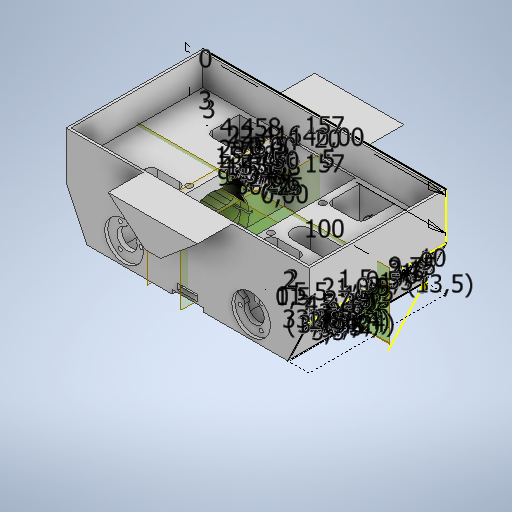
# Autodesk Inventor part: low_part
Saved by Autodesk Inventor 2025 (Build 290162000, 162)
## iProperties
Created: 2026-06-26
Part Number: low_part
Material: Типовые
Document SubType Name: Sheet Metal
Designer: garin
Density: 1 g/cm^3
Appearance: По умолчанию
Sheet Metal Rule: По умолчанию
Mass: 239.505 g
Surface Area: 434.405 cm^2
Volume: 239.505 cm^3
Author: garin
Autodesk Inventor part; units mm, degrees
(part 1 of 2)
ref_plane "YZ Plane" through (0, 0, 0) normal (1, 0, 0) x (0, 1, 0)
ref_plane "XZ Plane" through (0, 0, 0) normal (0, 1, 0) x (-1, 0, 0)
ref_plane "XY Plane" through (0, 0, 0) normal (0, 0, 1) x (1, 0, 0)
sketch "Эскиз2" plane through (0, 0, 0) normal (0, 0, 1) x (1, 0, 0)
  line L0 (0, 0) -> (-78.5, 0) construction
  line L1 (-78.5, 0) -> (78.5, 0)
  line L2 (0, 0) -> (-50, 0) construction
  line L3 (-50, 0) -> (-50, -28.5) construction
  line L4 (-50, -28.5) -> (-78.5, 0)
  line L5 (-50, -28.5) -> (50, -28.5)
  line L6 (50, -28.5) -> (78.5, 0)
  line L7 (-50, -28.5) -> (-45.542, -28.5) construction
  line L8 (-45.542, -28.5) -> (-45.542, -22.152) construction
  line L9 (-45.542, -22.152) -> (-50, -22.152) construction
  line L10 (-50, -22.152) -> (-50, -28.5) construction
  line L11 (-45.542, -22.152) -> (-45.542, -6.564) construction
  arc A0 (-45.542, -22.152) -> (-45.542, -6.564) centre (-50.0424, -14.358) ccw construction
  circle A1 centre (-45.542, -22.152) radius 1.3
  line L12 (-45.542, -22.152) -> (-32.0424, -14.358) construction
  line L13 (-45.542, -22.152) -> (-29.954, -22.152) construction
  circle A2 centre (-32.0424, -14.358) radius 1.3
  circle A3 centre (-45.542, -6.564) radius 1.3
  line L14 (-45.542, -6.564) -> (-32.0424, -14.358) construction
  circle A4 centre (-41.0424, -14.358) radius 12.5
  circle A5 centre (-41.0424, -14.358) radius 6.5
  line L15 (-41.0424, -14.358) -> (-41.0424, -26.858) construction
  line L16 (-41.0424, -14.358) -> (-34.7924, -25.1833) construction
  line L17 (-41.0424, -14.358) -> (-30.2171, -20.608) construction
  line L18 (-78.5, 0) -> (-75.5, 0) construction
  line L19 (-50, -28.5) -> (-47, -28.5) construction
  line L20 (-75.5, 0) -> (-47, -28.5)
  line L21 (-78.5, 0) -> (-75.5, 0) construction
  line L22 (-75.5, 0) -> (-75.5, -3) construction
  line L23 (-75.5, -3) -> (-78.5, -3) construction
  line L24 (-78.5, -3) -> (-78.5, 0) construction
  line L25 (-50, -28.5) -> (-50, -25.5) construction
  line L26 (-50, -28.5) -> (-47, -28.5) construction
  line L27 (-75.5, -3) -> (75.5, -3)
  line L28 (-75.5, -3) -> (75.5, -3) construction
  line L29 (0, 0) -> (0, -28.5) construction
  line L30 (75.5, 0) -> (47, -28.5)
  line L31 (-50, -25.5) -> (50, -25.5)
  line L32 (-50, -25.5) -> (50, -25.5) construction
  circle A6 centre (45.542, -22.152) radius 1.3
  circle A7 centre (32.0424, -14.358) radius 1.3
  circle A8 centre (45.542, -6.564) radius 1.3
  circle A9 centre (41.0424, -14.358) radius 12.5
  circle A10 centre (41.0424, -14.358) radius 6.5
  line L33 (41.0424, -14.358) -> (41.0424, -26.858) construction
  line L34 (41.0424, -14.358) -> (30.2171, -20.608) construction
  line L35 (-41.0424, -14.358) -> (-22.0786, -14.358) construction
  line L36 (-41.0424, -14.358) -> (-41.0424, -1.858)
  line L37 (-41.0424, -14.358) -> (-30.2171, -8.108)
  line L38 (41.0424, -14.358) -> (30.2171, -8.108)
  line L39 (41.0424, -14.358) -> (41.0424, -1.858)
  line L40 (-45.542, -6.564) -> (-50, -6.564) construction
  line L41 (-50, -6.564) -> (-50, 0) construction
  line L42 (-50, 0) -> (-45.542, 0) construction
  line L43 (-45.542, 0) -> (-45.542, -6.564) construction
  line L44 (-50, -25.5) -> (-27.584, -25.5)
  line L45 (-27.584, -25.5) -> (-27.584, 0)
  line L46 (-27.584, 0) -> (-50, 0)
  line L47 (-50, 0) -> (-50, -25.5)
  line L48 (27.584, -25.5) -> (27.584, 0)
  line L49 (50, 0) -> (50, -25.5)
  line L50 (-50, -28.5) -> (-65, -28.5)
  line L51 (-65, -28.5) -> (-78.5, 0)
  line L52 (-65, -28.5) -> (-62, -28.5)
  line L53 (-62, -28.5) -> (-75.5, 0)
  line L54 (-50, -25.5) -> (-63.4211, -25.5)
  line L55 (50, -28.5) -> (65, -28.5)
  line L56 (65, -28.5) -> (78.5, 0)
  line L57 (65, -28.5) -> (62, -28.5)
  line L58 (62, -28.5) -> (75.5, 0)
  point P0 (-72.5, -3)
  point P1 (72.5, -3)
  point P2 (-41.0424, -25.5)
  point P3 (-41.0424, -20.858)
  point P4 (-35.4132, -17.608)
  point P5 (-30.2171, -20.608)
  point P6 (-35.3762, -25.5)
  point P7 (35.3762, -25.5)
  point P8 (30.2171, -20.608)
  point P9 (35.4132, -17.608)
  point P10 (41.0424, -20.858)
  point P11 (41.0424, -25.5)
  point P12 (47, -28.5)
  point P13 (46.7086, -25.5)
  point P14 (41.0424, -26.858)
  point P15 (-46.7086, -25.5)
  point P16 (35.8226, -3)
  point P17 (41.0424, -3)
  point P18 (41.0424, -7.858)
  point P19 (35.4132, -11.108)
  point P20 (30.2171, -8.108)
  point P21 (-35.8226, -3)
  point P22 (-30.2171, -8.108)
  point P23 (-35.4132, -11.108)
  point P24 (-41.0424, -7.858)
  point P25 (-41.0424, -3)
  dimension "d0" = 78.5
  dimension "d1" = 157
  dimension "d2" = 50
  dimension "d3" = 28.5
  dimension "d4" = 100
  dimension "d15" = 4.458
  dimension "d16" = 6.348
  dimension "d17" = 15.588
  dimension "d18" = 9
  dimension "d19" = 2.6
  dimension "d20" = 15.588
  dimension "d21" = 30
  dimension "d22" = 2.6
  dimension "d23" = 2.6
  dimension "d24" = 25
  dimension "d25" = 13
  dimension "d26" = 12.5
  dimension "d29" = 30
  dimension "d31" = 3
  dimension "d32" = 3
  dimension "d33" = 3
  dimension "d34" = 90
  dimension "d35" = 0
  dimension "d36" = 0
  dimension "d48" = 4.458
  dimension "d49" = 22.416
  dimension "d151" = 15
  dimension "d152" = 3
  dimension "d153" = 15
  dimension "d154" = 3
  constraints: 118 end point, 17 symmetric about line, 13 point on line, 12 horizontal, 11 centre point, 9 parallel, 6 coincident, 5 perpendicular, 4 equal length, 3 point on circle, 3 vertical, 1 midpoint, 9 other
  measures "d0" distance of L0.start L0.end
  measures "d1" distance of L0.end L1.end
  measures "d2" distance of L0.start L2.end
  measures "d3" distance of L2.end L3.end
  measures "d4" distance of L3.end L5.end
  measures "d15" distance of L9.end L8.end
  measures "d16" distance of L8.end L7.end
  measures "d17" distance of L8.end L11.end
  measures "d18" radius of A0
  measures "d19" diameter of A1
  measures "d20" distance of L12.start L12.end
  measures "d21" angle of L13 L12
  measures "d22" diameter of A2
  measures "d23" diameter of A3
  measures "d24" diameter of A4
  measures "d25" diameter of A5
  measures "d26" distance of L15.start L15.end
  measures "d31" distance of L0.end L18.end
  measures "d32" distance of L3.end L19.end
  measures "d33" distance of L21.end L22.end
  measures "d34" angle of L26 L25
  measures "d35" distance between parallel lines of L27 L28
  measures "d36" distance between parallel lines of L31 L32
  measures "d48" distance of L41.end L42.end
  measures "d49" distance of L46.end L45.end
  measures "d151" distance of L3.end L50.end
  measures "d152" distance of L50.end L52.end
  measures "d153" distance of L5.end L55.end
  measures "d154" distance of L55.end L57.end
extrude "Выдавливание1" add sketch "Эскиз2" along normal blind 88.4 contours L1 L53 L27 L4 | L4 L53 L50 L51 | L1 L47 L27 L20 | L20 L27 L53 | L27 L53 L4 | L1 L45 L27 A4 L47 | L27 L47 A4 L20 | L20 L54 L4 L53 L27 | L4 L54 L53 | L53 L54 L4 L50 | L1 L48 L27 L45 | L27 A4 L47 | L31 A4 A9 L30 L5 L20 | L47 A4 L31 | L20 L5 L4 L54 | L1 L49 L27 A9 L48 | L45 L31 A4 L27 | L27 L48 L31 L45 | L27 L36 A5 L37 A4 L31 L47 | A4 L36 L27 | L47 A4 | L31 A4 | L1 L30 L27 L49 | L27 A9 L31 L48 | L27 L36 A4 | A4 L37 A5 L36 L27 | L30 L27 L58 L6 L5 | L58 L27 L30 | L1 L6 L27 L58 | L49 A9 L27 | L27 L30 L49 A9 | A9 L39 L27 | L27 L39 A10 L38 A9 | L36 L37 A5 | A5 L37 L36 | L6 L58 L55 | L31 A9 L49 | L56 L55 L58 L6 | L27 L6 L58 | A9 L49 L31 L38 A10 L39 L27 | L27 L39 A9 | A9 L49 | L31 A9 | L39 L38 A10 | A10 L38 L39 | A1 | A2 | A3 | A6 | A7 | A8
extrude "Выдавливание2" cut sketch "Эскиз2" along normal blind 5 contours A4 L37 A5 L36 L27 | L27 L39 A10 L38 A9 | L36 L37 A5 | A5 L37 L36 | L39 L38 A10 | A10 L38 L39 | A1 | A2 | A3 | A6 | A7 | A8
extrude "Выдавливание4" cut sketch "Эскиз2" along normal blind 2 contours L27 L36 A5 L37 A4 L31 L47 | A4 L36 L27 | L47 A4 | L31 A4 | L27 L36 A4 | A4 L37 A5 L36 L27 | A9 L39 L27 | L27 L39 A10 L38 A9 | L36 L37 A5 | A5 L37 L36 | A9 L49 L31 L38 A10 L39 L27 | L27 L39 A9 | A9 L49 | L31 A9 | L39 L38 A10 | A10 L38 L39 | A1 | A2 | A3 | A6 | A7 | A8
fillet "Сопряжение1" radius 2 4 edges at (35.4132, -11.108, 3.5) (41.0424, -7.858, 3.5) (-35.4132, -11.108, 3.5) (-41.0424, -7.858, 3.5)
extrude "Выдавливание6" cut sketch "Эскиз2" along normal blind 21.5 from surface at 5 contours L1 L45 L27 A4 L47 | L27 A4 L47 | L47 A4 L31 | L1 L49 L27 A9 L48 | L45 L31 A4 L27 | L27 L36 A5 L37 A4 L31 L47 | A4 L36 L27 | L27 A9 L31 L48 | L27 L36 A4 | A4 L37 A5 L36 L27 | L49 A9 L27 | A9 L39 L27 | L27 L39 A10 L38 A9 | L36 L37 A5 | A5 L37 L36 | L31 A9 L49 | A9 L49 L31 L38 A10 L39 L27 | L27 L39 A9 | L39 L38 A10 | A10 L38 L39 | A1 | A2 | A3 | A6 | A7 | A8
fillet "Сопряжение2" radius 4 4 edges at (50, -12.75, 26.5) (27.584, -12.75, 26.5) (-27.584, -12.75, 26.5) (-50, -12.75, 26.5)
ref_plane "РабПлоскость1" through (0, 0, 44.2) normal (0, 0, -1) x (-1, 0, 0)
mirror "Зеркальное отражение2" about plane through (0, 0, 44.2) normal (0, 0, -1) of "Выдавливание2", "Выдавливание6", "Сопряжение2", "Выдавливание4", "Сопряжение1"
sketch "Эскиз4" plane through (-78.5, 0, 0) normal (0, 1, 0) x (1, 0, 0)
  line L0 (78.5, 0) -> (78.5, -86) construction
  line L1 (28.5, -86) -> (128.5, -86) projected
  line L2 (0, 0) -> (0, -88.4) projected
  line L3 (0, -44.2) -> (157, -44.2) construction
  line L4 (157, 0) -> (157, -88.4) projected
  line L5 (78.5, -44.2) -> (101.4, -44.2) construction
  line L6 (101.4, -44.2) -> (101.4, -3) construction
  line L7 (101.4, -3) -> (78.5, -3) construction
  line L8 (78.5, -3) -> (78.5, -44.2) construction
  line L9 (101.4, -3) -> (55.6, -3)
  line L10 (55.6, -3) -> (55.6, -85.4)
  line L11 (55.6, -85.4) -> (101.4, -85.4)
  line L12 (101.4, -85.4) -> (101.4, -3)
  dimension "d53" = 22.9
  dimension "d54" = 41.2
  dimension "d55" = 45.8
  dimension "d56" = 82.4
  constraints: 20 end point, 4 midpoint, 4 parallel, 2 horizontal, 2 perpendicular
  measures "d53" distance of L7.end L6.end
  measures "d54" distance of L6.end L5.end
  measures "d55" distance of L11.end L10.end
  measures "d56" distance of L10.end L9.end
extrude "Выдавливание7" cut sketch "Эскиз4" against normal blind 28.5
sketch "Эскиз5" plane through (-78.5, 0, 0) normal (0, 1, 0) x (1, 0, 0)
  line L0 (0, 0) -> (157, 0)
  line L1 (157, 0) -> (157, -88.4)
  line L2 (157, -88.4) -> (0, -88.4)
  line L3 (0, -88.4) -> (0, 0)
  line L4 (55.6, -3) -> (101.4, -3) projected
  line L5 (55.6, -3) -> (55.6, -83) projected
  line L6 (101.4, -3) -> (55.6, -3)
  line L7 (55.6, -3) -> (55.6, -83)
  line L8 (55.6, -83) -> (101.4, -83)
  line L9 (101.4, -83) -> (101.4, -3)
  line L10 (104.4, 0) -> (52.6, 0)
  line L11 (52.6, 0) -> (52.6, -86)
  line L12 (52.6, -86) -> (104.4, -86)
  line L13 (104.4, -86) -> (104.4, 0)
  line L14 (3, -85.4) -> (154, -85.4)
  line L15 (154, -85.4) -> (154, -3)
  line L16 (154, -3) -> (3, -3)
  line L17 (3, -3) -> (3, -85.4)
  line L18 (104.4, 0) -> (106.084, 0)
  line L19 (106.084, 0) -> (106.084, -88.4)
  line L20 (106.084, -88.4) -> (104.4, -88.4)
  line L21 (104.4, -88.4) -> (104.4, 0)
  line L22 (52.6, 0) -> (50.916, 0)
  line L23 (50.916, 0) -> (50.916, -88.4)
  line L24 (50.916, -88.4) -> (52.6, -88.4)
  line L25 (52.6, -88.4) -> (52.6, 0)
  line L26 (50.916, 0) -> (52.916, 0) construction
  line L27 (0, -44.2) -> (157, -44.2) construction
  line L28 (78.5, -86) -> (78.5, 0) construction
  arc A0 (28.5, -22.5) -> (32.5, -26.5) centre (32.5, -22.5) ccw projected
  line L29 (46.916, -26.5) -> (32.5, -26.5) projected
  arc A1 (46.916, -26.5) -> (50.916, -22.5) centre (46.916, -22.5) ccw projected
  line L30 (50.916, -5) -> (50.916, -22.5) projected
  line L31 (50.916, -5) -> (28.5, -5) projected
  line L32 (28.5, -5) -> (28.5, -22.5) projected
  arc A2 (32.5, -61.9) -> (28.5, -65.9) centre (32.5, -65.9) ccw projected
  line L33 (28.5, -83.4) -> (28.5, -65.9) projected
  line L34 (50.916, -83.4) -> (28.5, -83.4) projected
  line L35 (50.916, -83.4) -> (50.916, -65.9) projected
  arc A3 (50.916, -65.9) -> (46.916, -61.9) centre (46.916, -65.9) ccw projected
  line L36 (46.916, -61.9) -> (32.5, -61.9) projected
  arc A4 (110.084, -61.9) -> (106.084, -65.9) centre (110.084, -65.9) ccw projected
  line L37 (106.084, -83.4) -> (106.084, -65.9) projected
  line L38 (128.5, -83.4) -> (106.084, -83.4) projected
  line L39 (128.5, -83.4) -> (128.5, -65.9) projected
  arc A5 (128.5, -65.9) -> (124.5, -61.9) centre (124.5, -65.9) ccw projected
  line L40 (124.5, -61.9) -> (110.084, -61.9) projected
  arc A6 (106.084, -22.5) -> (110.084, -26.5) centre (110.084, -22.5) ccw projected
  line L41 (124.5, -26.5) -> (110.084, -26.5) projected
  arc A7 (124.5, -26.5) -> (128.5, -22.5) centre (124.5, -22.5) ccw projected
  line L42 (128.5, -5) -> (128.5, -22.5) projected
  line L43 (128.5, -5) -> (106.084, -5) projected
  line L44 (106.084, -5) -> (106.084, -22.5) projected
  line L45 (46.916, -61.9) -> (55.6, -61.9) construction
  arc A8 (50.916, -65.9) -> (46.916, -61.9) centre (46.916, -65.9) ccw construction
  line L46 (46.916, -26.5) -> (55.6, -26.5) construction
  line L47 (55.6, -61.9) -> (52.1, -61.9) construction
  line L48 (52.1, -61.9) -> (52.1, -60.9) construction
  line L49 (52.1, -60.9) -> (55.6, -60.9) construction
  line L50 (55.6, -60.9) -> (55.6, -61.9) construction
  circle A9 centre (52.1, -60.9) radius 2.1
  circle A10 centre (52.1, -27.5) radius 2.1
  circle A11 centre (104.9, -60.9) radius 2.1
  circle A12 centre (104.9, -27.5) radius 2.1
  line L51 (101.4, -83) -> (55.6, -83)
  line L52 (55.6, -83) -> (55.6, -85.4)
  line L53 (55.6, -85.4) -> (101.4, -85.4)
  line L54 (101.4, -85.4) -> (101.4, -83)
  point P0 (50.916, -65.9)
  point P1 (50.916, -22.5)
  point P2 (50.916, -83.4)
  point P3 (106.084, -83.4)
  dimension "d59" = 157
  dimension "d60" = 88.4
  dimension "d61" = 3
  dimension "d62" = 3
  dimension "d63" = 1.684
  dimension "d64" = 1.684
  dimension "d72" = 3.5
  dimension "d73" = 1
  dimension "d74" = 4.2
  constraints: 74 end point, 16 parallel, 10 perpendicular, 7 horizontal, 5 point on line, 4 centre point, 3 midpoint, 3 symmetric about line, 3 tangent, 1 coincident, 1 vertical, 9 other
  measures "d59" distance of L1.end L2.end
  measures "d60" distance of L0.end L1.end
  measures "d61" distance between parallel lines of L9 L13
  measures "d62" distance between parallel lines of L2 L14
  measures "d63" distance of L19.end L20.end
  measures "d64" distance of L24.end L23.end
  measures "d72" distance of L48.end L49.end
  measures "d73" distance of L47.end L48.end
  measures "d74" diameter of A9
extrude "Выдавливание8" add sketch "Эскиз5" along normal blind 10.2 contours L0 L23 L16 L17 L14 L2 L3 | L0 L11 L16 L23 | L0 L13 L16 L4 L11 | L23 L31 L32 A0 L29 A1 A10 A9 A3 L36 A2 L33 L34 L14 L17 L16 | L16 L11 A10 L23 | L23 L14 L11 L25 L2 | L0 L19 L16 L13 | L16 L5 L52 L14 L11 A9 A10 | L25 L12 L21 L2 | L23 A9 L11 L14 | L0 L1 L2 L19 L14 L15 L16 | L16 L19 A12 L13 | L13 A12 A11 L14 L54 L9 L16 | L21 L13 L14 L19 L2 | L11 L14 L13 L12 | L16 L15 L14 L19 L38 L39 A5 L40 A4 A11 A12 A6 L41 A7 L42 L43 | L11 A9 L23 A10 | A12 L19 A11 L13 | L14 L13 A11 L19
sketch "Эскиз9" plane through (-65, -28.5, 0) normal (0, -1, 0) x (1, 0, 0)
  line L0 (130, 88.4) -> (143.5, 88.4) construction
  line L1 (0, 0) -> (130, 0) projected
  line L2 (143.5, 88.4) -> (130, 88.4) construction
  line L3 (130, 88.4) -> (130, 0) construction
  line L4 (130, 0) -> (143.5, 0) construction
  line L5 (143.5, 0) -> (143.5, 88.4) construction
  line L6 (130, 44.2) -> (87.9, 44.2) construction
  line L7 (87.9, 85.4) -> (87.9, 3) construction
  line L8 (130, 44.2) -> (87.9, 44.2) construction
  line L9 (87.9, 44.2) -> (87.9, 46.2) construction
  line L10 (87.9, 46.2) -> (130, 46.2) construction
  line L11 (130, 46.2) -> (130, 44.2) construction
  line L12 (130, 44.2) -> (87.9, 44.2) construction
  line L13 (87.9, 44.2) -> (87.9, 42.2) construction
  line L14 (87.9, 42.2) -> (130, 42.2) construction
  line L15 (130, 42.2) -> (130, 44.2) construction
  line L16 (130, 42.2) -> (127, 42.2) construction
  line L17 (127, 42.2) -> (106, 42.2)
  line L18 (106, 42.2) -> (106, 21.2)
  line L19 (106, 21.2) -> (127, 21.2)
  line L20 (127, 21.2) -> (127, 42.2)
  line L21 (127, 42.2) -> (124.364, 42.2) construction
  line L22 (124.364, 42.2) -> (124.364, 39.414) construction
  line L23 (124.364, 39.414) -> (127, 39.414) construction
  line L24 (127, 39.414) -> (127, 42.2) construction
  circle A0 centre (124.364, 39.414) radius 2
  line L25 (127, 42.2) -> (127, 46.2) construction
  line L26 (130, 46.2) -> (96.5, 46.2)
  line L27 (96.5, 46.2) -> (96.5, 57.2)
  line L28 (96.5, 57.2) -> (130, 57.2)
  line L29 (130, 57.2) -> (130, 46.2)
  line L30 (130, 46.2) -> (124.5, 46.2)
  line L31 (124.5, 46.2) -> (124.5, 57.2)
  line L32 (124.5, 57.2) -> (130, 57.2)
  line L33 (130, 57.2) -> (130, 46.2)
  line L34 (96.5, 57.2) -> (102, 57.2)
  line L35 (102, 57.2) -> (102, 46.2)
  line L36 (102, 46.2) -> (96.5, 46.2)
  line L37 (96.5, 46.2) -> (96.5, 57.2)
  arc A1 (124.5, 46.2) -> (124.5, 57.2) centre (124.5, 51.7) ccw
  arc A2 (102, 57.2) -> (102, 46.2) centre (102, 51.7) ccw
  circle A3 centre (102, 51.7) radius 2.1
  circle A4 centre (124.5, 51.7) radius 2.1
  line L38 (124.364, 39.414) -> (108.636, 39.414) construction
  circle A5 centre (108.636, 39.414) radius 2
  line L39 (124.5, 51.7) -> (117.5, 51.7) construction
  line L40 (124.5, 51.7) -> (131.5, 51.7) construction
  line L41 (102, 51.7) -> (109, 51.7) construction
  circle A6 centre (117.5, 51.7) radius 3
  circle A7 centre (109, 51.7) radius 3
  circle A8 centre (117.5, 51.7) radius 3.5 construction
  line L42 (122.4, 51.7) -> (121, 51.7) construction
  line L43 (121.7, 51.7) -> (121.7, 46.2)
  line L44 (121.7, 51.7) -> (121.7, 57.2)
  line L45 (113.25, 46.2) -> (113.25, 57.2) construction
  line L46 (104.8, 51.7) -> (104.8, 46.2)
  line L47 (104.8, 51.7) -> (104.8, 57.2)
  arc A9 (124.5, 45.7) -> (124.5, 57.7) centre (124.5, 51.7) ccw
  arc A10 (102, 57.7) -> (102, 45.7) centre (102, 51.7) ccw
  line L48 (124.5, 57.7) -> (102, 57.7)
  line L49 (124.5, 45.7) -> (102, 45.7)
  line L50 (121.7, 46.2) -> (121.7, 45.7)
  line L51 (121.7, 57.2) -> (121.7, 57.7)
  line L52 (104.8, 57.2) -> (104.8, 57.7)
  line L53 (104.8, 46.2) -> (104.8, 45.7)
  line L54 (106, 21.2) -> (107.5, 21.2)
  line L55 (107.5, 21.2) -> (125.5, 21.2)
  line L56 (125.5, 21.2) -> (125.5, 24.2)
  line L57 (125.5, 24.2) -> (107.5, 24.2)
  line L58 (107.5, 24.2) -> (107.5, 21.2)
  point P0 (65, 0)
  point P1 (124.5, 46.2)
  point P2 (125.5, 21.2)
  dimension "d173" = 4.2
  dimension "d181" = 7
  dimension "d155" = 13.5
  dimension "d156" = 88.4
  dimension "d157" = 2
  dimension "d158" = 2
  dimension "d159" = 3
  dimension "d160" = 21
  dimension "d161" = 21
  dimension "d162" = 2.636
  dimension "d163" = 2.786
  dimension "d164" = 4
  dimension "d168" = 33.5
  dimension "d169" = 11
  dimension "d170" = 5.5
  dimension "d171" = 5.5
  dimension "d172" = 4.2
  dimension "d174" = 15.728
  dimension "d175" = 4
  dimension "d176" = 7
  dimension "d177" = 180
  dimension "d178" = 7
  dimension "d179" = 6
  dimension "d180" = 6
  dimension "d182" = 0.5
  dimension "d183" = 0.5
  dimension "d196" = 1.5
  dimension "d197" = 18
  dimension "d198" = 3
  constraints: 112 end point, 19 parallel, 19 point on line, 13 horizontal, 13 perpendicular, 9 centre point, 8 point on circle, 7 coincident, 6 midpoint, 6 tangent, 3 symmetric about line, 2 horizontal alignment, 1 collinear, 4 other
  measures "d155" distance of L4.end L1.end
  measures "d156" distance of L1.end L2.end
  measures "d157" distance of L8.end L9.end
  measures "d158" distance of L13.end L12.end
  measures "d159" distance of L14.end L16.end
  measures "d160" distance of L19.end L18.end
  measures "d161" distance of L18.end L17.end
  measures "d162" distance of L23.end L22.end
  measures "d163" distance of L22.end L21.end
  measures "d164" diameter of A0
  measures "d168" distance of L27.end L28.end
  measures "d169" distance of L26.end L27.end
  measures "d170" distance of L31.end L32.end
  measures "d171" distance of L35.end L36.end
  measures "d172" diameter of A3
  measures "d174" distance of L38.start L38.end
  measures "d175" diameter of A5
  measures "d176" distance of L39.start L39.end
  measures "d177" angle of L39 L40
  measures "d178" distance of L41.start L41.end
  measures "d179" diameter of A6
  measures "d180" diameter of A7
  measures "d182" radial gap between concentric circles of A1 A9
  measures "d183" radial gap between concentric circles of A2 A10
  measures "d196" distance of L18.end L54.end
  measures "d197" distance of L57.end L56.end
  measures "d198" distance of L56.end L55.end
extrude "Выдавливание17" cut sketch "Эскиз9" along normal blind 30 from surface at -38.7 contours L26 A9 L49 L50 | A1 L29 A9 L26 | L26 L43 L44 L28 L31 A4 | L31 A4 A1 | L50 L49 L53 L26 | L26 L46 L47 L28 L44 L43 | A4 L31 | L31 A4 | A1 L28 A9 L29 | L29 A9 | L53 L49 A10 L26 | L26 L35 A3 L28 L47 L46 | L28 L51 L48 A9 | A2 L35 A3 | L26 A10 L27 A2 | L28 L52 L48 L51 | A3 L35 | L35 A3 | L27 A10 | L27 A10 L28 A2 | L28 A10 L48 L52 | A6 | A7
extrude "Выдавливание18" cut sketch "Эскиз9" along normal blind 2 from surface at -8.7 contours L50 L49 L53 L26 | L26 L46 L47 L28 L44 L43 | L28 L52 L48 L51 | A6 | A7
extrude "Выдавливание19" cut sketch "Эскиз9" along normal blind 8.7 from surface at -8.7 contours A6 | A7
extrude "Выдавливание20" cut sketch "Эскиз9" along normal blind 6.7 from surface at -8.7 contours A4 L31 | L31 A4 | A3 L35 | L35 A3
extrude "Выдавливание21" cut sketch "Эскиз9" against normal blind 1.5 contours L20 L19 L56 L57 L58 L18 L17 | L19 L58 L57 L56 | A0 | A5
extrude "Выдавливание22" cut sketch "Эскиз9" against normal blind 6 from surface at -1.5 contours A0 | A5
extrude "Выдавливание23" cut sketch "Эскиз9" against normal blind 6 contours L19 L58 L57 L56
sketch "Эскиз10" plane through (65, -28.5, 88.4) normal (0.9037378, -0.4280863, 0) x (0, 0, -1)
  line L0 (88.4, 31.5357) -> (0, 31.5357) projected
  line L1 (88.4, -55.6512) -> (88.4, 0) projected
  line L2 (0, 31.5357) -> (88.4, 31.5357)
  line L3 (88.4, 31.5357) -> (88.4, 0)
  line L4 (88.4, 0) -> (0, 0)
  line L5 (0, 0) -> (0, 31.5357)
  line L6 (44.2, 31.5357) -> (44.2, 0) construction
  line L7 (12.2, 28.0357) -> (74.2, 28.0357)
  line L8 (74.2, 28.0357) -> (74.2, 19.0357)
  line L9 (74.2, 19.0357) -> (12.2, 19.0357)
  line L10 (12.2, 19.0357) -> (12.2, 28.0357)
  line L11 (43.2, 28.0357) -> (43.2, 19.0357)
  line L12 (12.2, 19.0357) -> (14, 19.0357) construction
  line L13 (14, 19.0357) -> (14, 21.5357) construction
  line L14 (14, 21.5357) -> (12.2, 21.5357) construction
  line L15 (12.2, 21.5357) -> (12.2, 19.0357) construction
  circle A0 centre (14, 21.5357) radius 1.75
  line L16 (14, 21.5357) -> (14, 25.5357) construction
  circle A1 centre (14, 25.5357) radius 1.75
  line L17 (74.2, 19.0357) -> (64.45, 19.0357) construction
  line L18 (74.2, 21.1357) -> (74.2, 19.0357) construction
  line L19 (12.2, 28.0357) -> (39.7, 28.0357) construction
  line L20 (39.7, 28.0357) -> (48.7, 28.0357) construction
  line L21 (48.7, 28.0357) -> (48.7, 19.0357)
  line L22 (48.7, 19.0357) -> (39.7, 19.0357) construction
  line L23 (39.7, 19.0357) -> (39.7, 28.0357)
  line L24 (74.7, 28.5357) -> (11.7, 28.5357)
  line L25 (11.7, 28.5357) -> (11.7, 18.5357)
  line L26 (11.7, 18.5357) -> (74.7, 18.5357)
  line L27 (74.7, 18.5357) -> (74.7, 28.5357)
  line L28 (48.7, 28.0357) -> (49.2, 28.0357) construction
  line L29 (49.2, 28.0357) -> (49.2, 28.5357) construction
  line L30 (49.2, 28.5357) -> (48.7, 28.5357) construction
  line L31 (48.7, 28.5357) -> (48.7, 28.0357) construction
  line L32 (49.2, 28.5357) -> (49.2, 18.5357)
  line L33 (44.2, 28.0357) -> (44.2, 19.0357) construction
  line L34 (39.2, 28.5357) -> (39.2, 18.5357)
  line L35 (44.2, 28.5357) -> (44.2, 28.0357) construction
  line L36 (44.2, 31.5357) -> (44.2, 28.5357) construction
  line L37 (74.7, 28.5357) -> (82.7, 28.5357)
  line L38 (82.7, 28.5357) -> (82.7, 18.5357)
  line L39 (82.7, 18.5357) -> (74.7, 18.5357)
  line L40 (74.7, 18.5357) -> (74.7, 28.5357)
  line L41 (74.7, 28.5357) -> (68.7, 28.5357)
  line L42 (68.7, 28.5357) -> (68.7, 18.5357)
  line L43 (68.7, 18.5357) -> (74.7, 18.5357)
  line L44 (74.7, 18.5357) -> (74.7, 28.5357)
  line L45 (74.2, 28.0357) -> (64.45, 28.0357) construction
  line L46 (64.45, 28.0357) -> (64.45, 25.9357) construction
  line L47 (64.45, 25.9357) -> (74.2, 25.9357) construction
  line L48 (74.2, 25.9357) -> (74.2, 28.0357) construction
  circle A2 centre (64.45, 25.9357) radius 1.75
  line L49 (12.2, 28.0357) -> (15.85, 28.0357) construction
  line L50 (15.85, 28.0357) -> (15.85, 19.0357)
  line L51 (15.85, 19.0357) -> (12.2, 19.0357) construction
  line L52 (12.2, 19.0357) -> (12.2, 28.0357) construction
  line L53 (39.7, 28.0357) -> (37.2, 28.0357) construction
  line L54 (37.2, 28.0357) -> (37.2, 19.0357)
  line L55 (37.2, 19.0357) -> (39.7, 19.0357) construction
  line L56 (39.7, 19.0357) -> (39.7, 28.0357) construction
  line L57 (48.7, 28.0357) -> (50.2, 28.0357) construction
  line L58 (50.2, 28.0357) -> (50.2, 19.0357)
  line L59 (50.2, 19.0357) -> (48.7, 19.0357) construction
  line L60 (48.7, 19.0357) -> (48.7, 28.0357) construction
  line L61 (62.7, 25.9357) -> (62.7, 28.0357) construction
  line L62 (62.7, 28.0357) -> (61.2, 28.0357) construction
  line L63 (61.2, 28.0357) -> (61.2, 19.0357)
  line L64 (61.2, 19.0357) -> (62.7, 19.0357) construction
  line L65 (62.7, 19.0357) -> (62.7, 28.0357) construction
  line L66 (15.85, 19.0357) -> (15.85, 18.5357)
  line L67 (15.85, 28.0357) -> (15.85, 28.5357)
  line L68 (37.2, 28.0357) -> (37.2, 28.5357)
  line L69 (37.2, 19.0357) -> (37.2, 18.5357)
  line L70 (50.2, 28.0357) -> (50.2, 28.5357)
  line L71 (50.2, 19.0357) -> (50.2, 18.5357)
  line L72 (61.2, 28.0357) -> (61.2, 28.5357)
  line L73 (61.2, 19.0357) -> (61.2, 18.5357)
  point P0 (88.4, -2.0691)
  point P1 (44.2, 23.5357)
  point P2 (39.2, 28.5357)
  point P3 (39.2, 18.5357)
  point P4 (61.2, 19.0357)
  point P5 (61.2, 28.0357)
  point P6 (50.2, 28.0357)
  point P7 (37.2, 19.0357)
  point P8 (37.2, 28.0357)
  point P9 (15.85, 28.0357)
  point P10 (15.85, 19.0357)
  point P11 (37.2, 28.0357)
  point P12 (15.85, 28.0357)
  point P13 (37.2, 19.0357)
  point P14 (15.85, 19.0357)
  point P15 (61.2, 28.0357)
  point P16 (50.2, 28.0357)
  point P17 (61.2, 19.0357)
  dimension "d366" = 3.5
  dimension "d201" = 88.4
  dimension "d202" = 62
  dimension "d203" = 9
  dimension "d206" = 1.8
  dimension "d207" = 2.5
  dimension "d208" = 3.5
  dimension "d209" = 4
  dimension "d210" = 3.5
  dimension "d214" = 27.5
  dimension "d215" = 9
  dimension "d216" = 9
  dimension "d217" = 0.5
  dimension "d218" = 0.5
  dimension "d219" = 3
  dimension "d220" = 8
  dimension "d221" = 10
  dimension "d231" = 6
  dimension "d364" = 9.75
  dimension "d365" = 2.1
  dimension "d367" = 3.65
  dimension "d368" = 9
  dimension "d369" = 2.5
  dimension "d370" = 9
  dimension "d371" = 1.5
  dimension "d372" = 1.5
  dimension "d373" = 9
  constraints: 144 end point, 26 parallel, 22 point on line, 18 perpendicular, 13 horizontal, 7 midpoint, 3 coincident, 2 centre point, 2 symmetric about line, 2 vertical, 1 horizontal alignment, 5 other
  measures "d201" distance of L1.end L4.end
  measures "d202" distance of L8.end L9.end
  measures "d203" distance of L7.end L8.end
  measures "d206" distance of L14.end L13.end
  measures "d207" distance of L13.end L12.end
  measures "d208" diameter of A0
  measures "d209" distance of L16.start L16.end
  measures "d210" diameter of A1
  measures "d214" distance of L7.start L19.end
  measures "d215" distance of L21.end L22.end
  measures "d216" distance of L20.end L21.end
  measures "d217" distance between parallel lines of L7 L24
  measures "d218" distance of L30.end L29.end
  measures "d219" distance of L6.start L35.start
  measures "d220" distance of L38.end L39.end
  measures "d221" distance of L37.end L38.end
  measures "d231" distance of L43.end L42.end
  measures "d364" distance of L47.end L46.end
  measures "d365" distance of L46.end L45.end
  measures "d367" distance of L50.end L51.end
  measures "d368" distance of L49.end L50.end
  measures "d369" distance of L55.end L54.end
  measures "d370" distance of L54.end L53.end
  measures "d371" distance of L58.end L59.end
  measures "d372" distance of L64.end L63.end
  measures "d373" distance of L63.end L62.end
extrude "Выдавливание24" cut sketch "Эскиз10" against normal blind 6 contours L34 L24 L32 L7 | L7 L23 L9 L34 | L7 L11 L9 L23 | L9 L32 L26 L34 | L7 L21 L9 L11 | L7 L32 L9 L21
extrude "Выдавливание25" cut sketch "Эскиз10" against normal blind 10.2 from surface at -6 contours L10 L9 L66 L26 L25 L24 L67 L7 | L7 L50 L9 L10 | L67 L24 L68 L7 | L7 L54 L9 L50 | L68 L24 L34 L7 | L7 L34 L9 L54 | L9 L69 L26 L66 | L34 L24 L32 L7 | L7 L23 L9 L34 | L9 L34 L26 L69 | L7 L11 L9 L23 | L9 L32 L26 L34 | L7 L21 L9 L11 | L24 L70 L7 L32 | L7 L32 L9 L21 | L24 L72 L7 L70 | L7 L58 L9 L32 | L32 L9 L71 L26 | L24 L42 L7 L72 | L7 L63 L9 L58 | L71 L9 L73 L26 | L24 L27 L26 L42 L9 L8 L7 | L7 L42 L9 L63 | L73 L9 L42 L26 | L37 L38 L39 L27 | L7 L8 L9 L42 | A0 | A1 | A2
ref_plane "РабПлоскость4" through (71.7933, -0.1427, 49.2) normal (0, -1, 0) x (1, 0, 0)
sketch "Эскиз12" plane through (71.7933, -0.1427, 49.2) normal (0, -1, 0) x (1, 0, 0)
  line L0 (0, 27.5) -> (-4.2809, 27.5) projected
  line L1 (-13.499, -43.5) -> (-4.2809, -43.5) projected
  line L2 (0, 27.5) -> (-13.499, 27.5)
  line L3 (-13.499, 27.5) -> (-13.499, -43.5)
  line L4 (-13.499, -43.5) -> (0, -43.5)
  line L5 (0, -43.5) -> (0, 27.5)
  line L6 (-13.499, -43.5) -> (-11.286, -43.5)
  line L7 (-11.286, -43.5) -> (-11.286, 27.5)
  line L8 (-11.286, 27.5) -> (-13.499, 27.5)
  line L9 (-13.499, 27.5) -> (-13.499, -43.5)
  point P0 (-71.7933, -49.2)
  point P1 (-4.2809, -43.5)
  point P2 (-4.2809, 27.5)
  point P3 (-11.286, -43.5)
  dimension "d228" = 2.213
  constraints: 16 end point, 4 parallel, 2 horizontal, 2 perpendicular, 1 point on line
  measures "d228" distance of L8.end L7.end
extrude "Выдавливание26" cut sketch "Эскиз12" against normal blind 12 from surface at 0 contours L5 L4 L1 L7 L2 L0
extrude "Выдавливание27" cut sketch "Эскиз10" along normal blind 5 from surface at -6 contours A0 | A1 | A2
extrude "Выдавливание28" cut sketch "Эскиз10" along normal blind 5 from surface at -6 contours L24 L27 L26 L42 L9 L8 L7 | L37 L38 L39 L27 | L7 L8 L9 L42
sketch "Эскиз13" plane through (0, 0, 0) normal (0, 0, -1) x (-1, 0, 0)
  line L0 (0, 0) -> (0, -28.5) construction
  line L1 (-22.9, -28.5) -> (22.9, -28.5) construction
  line L2 (-10, -28.5) -> (10, -28.5)
  line L3 (10, -28.5) -> (10, -26)
  line L4 (10, -26) -> (-10, -26)
  line L5 (-10, -26) -> (-10, -28.5)
  line L6 (-6.4, -24.5) -> (6.4, -24.5)
  line L7 (6.4, -24.5) -> (6.4, -20.5)
  line L8 (6.4, -20.5) -> (-6.4, -20.5)
  line L9 (-6.4, -20.5) -> (-6.4, -24.5)
  line L10 (-10, -28.5) -> (10, -28.5) construction
  line L11 (10, -28.5) -> (10, -24.5) construction
  line L12 (10, -24.5) -> (-10, -24.5) construction
  line L13 (-10, -24.5) -> (-10, -28.5) construction
  line L14 (0, -20.5) -> (0, -24.5) construction
  dimension "d234" = 20
  dimension "d235" = 2.5
  dimension "d240" = 12.8
  dimension "d241" = 4
  dimension "d242" = 20
  dimension "d243" = 4
  constraints: 28 end point, 6 parallel, 5 midpoint, 3 horizontal, 3 perpendicular
  measures "d234" distance of L4.end L3.end
  measures "d235" distance of L3.end L2.end
  measures "d240" distance of L8.end L7.end
  measures "d241" distance of L7.end L6.end
  measures "d242" distance of L12.end L11.end
  measures "d243" distance of L11.end L10.end
extrude "Выдавливание29" cut sketch "Эскиз13" against normal blind 3
extrude "Выдавливание30" cut sketch "Эскиз13" along normal blind 3 from surface at -88.4
sketch "Эскиз14" plane through (-22.9, -28.5, 85.4) normal (1, 0, 0) x (0, 0, -1)
  line L0 (85.4, 38.7) -> (-3, 38.7) projected
  line L1 (-3, 38.7) -> (85.4, 38.7)
  line L2 (85.4, 38.7) -> (85.4, 0)
  line L3 (85.4, 0) -> (-3, 0)
  line L4 (-3, 0) -> (-3, 38.7)
  line L5 (41.2, 38.7) -> (41.2, 0) construction
  line L6 (41.2, 0) -> (41.2, 3) construction
  line L7 (41.2, 3) -> (39.9, 3) construction
  line L8 (39.9, 3) -> (39.9, 7.5) construction
  line L9 (39.9, 7.5) -> (41.2, 7.5) construction
  line L10 (41.2, 7.5) -> (41.2, 3) construction
  line L11 (39.9, 7.5) -> (54.4, 7.5) construction
  line L12 (39.9, 7.5) -> (54.4, 7.5) construction
  line L13 (39.9, 3) -> (54.4, 3)
  line L14 (54.4, 12) -> (39.9, 12)
  arc A0 (39.9, 12) -> (39.9, 3) centre (39.9, 7.5) ccw
  arc A1 (54.4, 3) -> (54.4, 12) centre (54.4, 7.5) ccw
  line L15 (35.4, 7.5) -> (35.425, 7.5) construction
  line L16 (35.425, 7.5) -> (35.425, 7.025) construction
  line L17 (35.425, 7.025) -> (35.4, 7.025) construction
  line L18 (35.4, 7.025) -> (35.4, 7.5) construction
  line L19 (35.425, 7.025) -> (32.65, 7.025)
  line L20 (32.65, 7.025) -> (32.65, 7.975)
  line L21 (32.65, 7.975) -> (35.425, 7.975)
  line L22 (35.425, 7.975) -> (35.425, 7.025)
  line L23 (39.9, 12.1) -> (54.4, 12.1)
  arc A2 (54.4, 2.9) -> (54.4, 12.1) centre (54.4, 7.5) ccw
  line L24 (54.4, 2.9) -> (39.9, 2.9)
  arc A3 (39.9, 12.1) -> (39.9, 2.9) centre (39.9, 7.5) ccw
  circle A4 centre (41.2, 7.5) radius 1.925
  line L25 (41.2, 12.1) -> (41.2, 15.1) construction
  line L26 (27.2, 27.1) -> (55.2, 27.1)
  line L27 (55.2, 27.1) -> (55.2, 15.1)
  line L28 (55.2, 15.1) -> (27.2, 15.1)
  line L29 (27.2, 15.1) -> (27.2, 27.1)
  line L30 (41.2, 27.1) -> (41.2, 15.1) construction
  line L31 (41.2, 7.5) -> (22.2, 7.5) construction
  line L32 (41.2, 7.5) -> (60.2, 7.5) construction
  line L33 (41.2, 7.5) -> (60.2, 7.5) construction
  line L34 (85.4, 0) -> (-3, 0) projected
  line L35 (27.2, 15.1) -> (42.5329, 15.1) construction
  line L36 (-3, 0) -> (1, 0) construction
  line L37 (1, 0) -> (16, 0) construction
  line L38 (16, 0) -> (16, 27.1) construction
  line L39 (1, 0) -> (1, 27.1) construction
  line L40 (27.2, 27.1) -> (20.2, 27.1)
  line L41 (20.2, 27.1) -> (4.7731, 8.7149)
  line L42 (21.0316, 0) -> (6.0316, 0)
  line L43 (4.7731, 8.7149) -> (4.7731, 1.7149)
  line L44 (4.7731, 1.7149) -> (3.783, 0)
  line L45 (4.7731, 1.7149) -> (6.7533, 1.7149) construction
  line L46 (27.2, 15.1) -> (55.2, 15.1) construction
  line L47 (55.2, 15.1) -> (55.2, 30.1) construction
  line L48 (55.2, 30.1) -> (27.2, 30.1) construction
  line L49 (27.2, 30.1) -> (27.2, 15.1) construction
  line L50 (27.2, 30.1) -> (27.2, 28.1) construction
  line L51 (27.2, 28.1) -> (26.2, 28.1) construction
  line L52 (26.2, 28.1) -> (26.2, 25.1) construction
  line L53 (26.2, 25.1) -> (27.2, 25.1) construction
  line L54 (27.2, 25.1) -> (27.2, 28.1) construction
  line L55 (27.2, 15.1) -> (27.2, 17.1) construction
  line L56 (27.2, 17.1) -> (26.2, 17.1) construction
  line L57 (26.2, 17.1) -> (26.2, 20.1) construction
  line L58 (26.2, 20.1) -> (27.2, 20.1) construction
  line L59 (27.2, 20.1) -> (27.2, 17.1) construction
  line L60 (27.2, 28.1) -> (26.2, 25.1)
  line L61 (26.2, 25.1) -> (26.2, 20.1)
  line L62 (26.2, 20.1) -> (27.2, 17.1)
  line L63 (27.2, 30.1) -> (29.2, 30.1) construction
  line L64 (29.2, 30.1) -> (32.2, 30.1) construction
  line L65 (32.2, 30.1) -> (32.2, 31.1) construction
  line L66 (32.2, 31.1) -> (29.2, 31.1) construction
  line L67 (29.2, 31.1) -> (29.2, 30.1) construction
  line L68 (29.2, 30.1) -> (32.2, 31.1)
  line L69 (37.2, 31.1) -> (40.2, 31.1) construction
  line L70 (40.2, 31.1) -> (40.2, 30.1) construction
  line L71 (40.2, 30.1) -> (37.2, 30.1) construction
  line L72 (37.2, 30.1) -> (37.2, 31.1) construction
  line L73 (27.2, 22.6) -> (55.2, 22.6) construction
  line L74 (55.2, 28.1) -> (56.2, 25.1)
  line L75 (56.2, 25.1) -> (56.2, 20.1)
  line L76 (56.2, 20.1) -> (55.2, 17.1)
  line L77 (53.2, 30.1) -> (50.2, 31.1)
  line L78 (50.2, 31.1) -> (45.2, 31.1)
  line L79 (45.2, 31.1) -> (42.2, 30.1)
  line L80 (29.2, 15.1) -> (32.2, 14.1)
  line L81 (32.2, 14.1) -> (37.2, 14.1)
  line L82 (37.2, 14.1) -> (40.2, 15.1)
  line L83 (50.2, 14.1) -> (45.2, 14.1)
  line L84 (53.2, 15.1) -> (50.2, 14.1)
  line L85 (45.2, 14.1) -> (42.2, 15.1)
  arc A5 (29.2, 30.1) -> (27.2, 28.1) centre (29.2, 28.1) ccw
  arc A6 (55.2, 28.1) -> (53.2, 30.1) centre (53.2, 28.1) ccw
  arc A7 (53.2, 15.1) -> (55.2, 17.1) centre (53.2, 17.1) ccw
  arc A8 (27.2, 17.1) -> (29.2, 15.1) centre (29.2, 17.1) ccw
  line L86 (32.2, 31.1) -> (37.2, 31.1)
  line L87 (37.2, 31.1) -> (40.2, 30.1)
  line L88 (40.2, 30.1) -> (42.2, 30.1)
  line L89 (40.2, 15.1) -> (42.2, 15.1)
  line L90 (45.1675, 13.9) -> (50.2325, 13.9)
  line L91 (50.2325, 13.9) -> (53.2332, 14.9003)
  arc A9 (53.2332, 14.9003) -> (55.3997, 17.0668) centre (53.2, 17.1) ccw
  line L92 (55.3997, 17.0668) -> (56.4, 20.0675)
  line L93 (56.4, 20.0675) -> (56.4, 25.1325)
  line L94 (56.4, 25.1325) -> (55.3997, 28.1332)
  arc A10 (55.3997, 28.1332) -> (53.2332, 30.2997) centre (53.2, 28.1) ccw
  line L95 (53.2332, 30.2997) -> (50.2325, 31.3)
  line L96 (50.2325, 31.3) -> (45.1675, 31.3)
  line L97 (45.1675, 31.3) -> (42.1675, 30.3)
  line L98 (42.1675, 30.3) -> (40.2325, 30.3)
  line L99 (40.2325, 30.3) -> (37.2325, 31.3)
  line L100 (37.2325, 31.3) -> (32.1675, 31.3)
  line L101 (32.1675, 31.3) -> (29.1668, 30.2997)
  arc A11 (29.1668, 30.2997) -> (27.0003, 28.1332) centre (29.2, 28.1) ccw
  line L102 (27.0003, 28.1332) -> (26, 25.1325)
  line L103 (26, 25.1325) -> (26, 20.0675)
  line L104 (26, 20.0675) -> (27.0003, 17.0668)
  arc A12 (27.0003, 17.0668) -> (29.1668, 14.9003) centre (29.2, 17.1) ccw
  line L105 (29.1668, 14.9003) -> (32.1675, 13.9)
  line L106 (32.1675, 13.9) -> (37.2325, 13.9)
  line L107 (37.2325, 13.9) -> (40.2325, 14.9)
  line L108 (40.2325, 14.9) -> (42.1675, 14.9)
  line L109 (42.1675, 14.9) -> (45.1675, 13.9)
  line L110 (3.783, 0) -> (18.783, 0)
  line L111 (4.7731, 8.7149) -> (19.7731, 8.7149) construction
  line L112 (19.7731, 5.6814) -> (19.7731, 3.0547)
  line L113 (19.1032, 0.5547) -> (18.783, 0)
  line L114 (27.2, 17.1) -> (21.7844, 10.9858)
  arc A13 (21.7844, 10.9858) -> (19.7731, 5.6814) centre (27.7731, 5.6814) ccw
  arc A14 (19.1032, 0.5547) -> (19.7731, 3.0547) centre (14.7731, 3.0547) ccw
  line L115 (55.2, 27.1) -> (62.2, 27.1)
  line L116 (62.2, 27.1) -> (77.6269, 8.7149)
  line L117 (77.6269, 8.7149) -> (77.6269, 1.7149)
  line L118 (77.6269, 1.7149) -> (78.617, 0)
  line L119 (62.6269, 5.6814) -> (62.6269, 3.0547)
  line L120 (63.2968, 0.5547) -> (63.617, 0)
  line L121 (55.2, 17.1) -> (60.6156, 10.9858)
  arc A15 (62.6269, 5.6814) -> (60.6156, 10.9858) centre (54.6269, 5.6814) ccw
  arc A16 (62.6269, 3.0547) -> (63.2968, 0.5547) centre (67.6269, 3.0547) ccw
  line L122 (27.2, 27.1) -> (27.2, 28.7)
  line L123 (27.2, 15.2902) -> (22.6827, 10.1901)
  arc A17 (22.6827, 10.1901) -> (20.9731, 5.6814) centre (27.7731, 5.6814) ccw
  line L124 (20.9731, 5.6814) -> (20.9731, 3.0547)
  arc A18 (20.1425, -0.0453) -> (20.9731, 3.0547) centre (14.7731, 3.0547) ccw
  line L125 (20.1425, -0.0453) -> (19.4758, -1.2)
  line L126 (19.4758, -1.2) -> (1.7045, -1.2)
  line L127 (1.7045, -1.2) -> (3.5731, 2.0365)
  line L128 (3.5731, 2.0365) -> (3.5731, 9.1517)
  line L129 (3.5731, 9.1517) -> (19.6404, 28.3)
  line L130 (19.6404, 28.3) -> (27.2, 28.3)
  line L131 (63.617, 0) -> (78.617, 0)
  line L132 (55.2, 15.2902) -> (59.7173, 10.1901)
  arc A19 (61.4269, 5.6814) -> (59.7173, 10.1901) centre (54.6269, 5.6814) ccw
  line L133 (61.4269, 5.6814) -> (61.4269, 3.0547)
  arc A20 (61.4269, 3.0547) -> (62.2575, -0.0453) centre (67.6269, 3.0547) ccw
  line L134 (62.2575, -0.0453) -> (62.9242, -1.2)
  line L135 (62.9242, -1.2) -> (80.6955, -1.2)
  line L136 (80.6955, -1.2) -> (78.8269, 2.0365)
  line L137 (78.8269, 2.0365) -> (78.8269, 9.1517)
  line L138 (78.8269, 9.1517) -> (62.7596, 28.3)
  line L139 (62.7596, 28.3) -> (55.2, 28.3)
  line L140 (26, 20.0675) -> (24.7, 20.0675) construction
  line L141 (24.7, 20.0675) -> (24.7, 12.4676) construction
  line L142 (24.7, 12.4676) -> (26, 12.4676) construction
  line L143 (26, 12.4676) -> (26, 20.0675) construction
  line L144 (24.7, 12.4676) -> (24.7, 0)
  line L145 (57.7, 12.4676) -> (57.7, 0)
  line L146 (3.5731, 9.1517) -> (2.5571, 9.1517) construction
  line L147 (2.5571, 9.1517) -> (2.5571, 0) construction
  line L148 (2.5571, 0) -> (3.5731, 0) construction
  line L149 (3.5731, 0) -> (3.5731, 9.1517) construction
  line L150 (3.5731, 9.1517) -> (2.5571, 7.9409)
  line L151 (2.5571, 7.9409) -> (2.5571, 0)
  line L152 (78.8269, 9.1517) -> (79.8429, 7.9409)
  line L153 (79.8429, 7.9409) -> (79.8429, 0)
  line L154 (35.525, 8.075) -> (32.55, 8.075)
  line L155 (32.55, 8.075) -> (32.55, 6.925)
  line L156 (32.55, 6.925) -> (35.525, 6.925)
  line L157 (35.525, 6.925) -> (35.525, 8.075)
  line L158 (47.15, 12.1) -> (47.15, 2.9) construction
  line L159 (58.775, 8.075) -> (61.75, 8.075)
  line L160 (61.75, 8.075) -> (61.75, 6.925)
  line L161 (61.75, 6.925) -> (58.775, 6.925)
  circle A21 centre (54.4, 7.5) radius 3.5
  circle A22 centre (54.4, 7.5) radius 3.6
  line L162 (41.2, 7.5) -> (24.2885, 0)
  line L163 (41.2, 7.5) -> (58.1115, 0)
  arc A23 (58.1115, 0) -> (24.2885, 0) centre (41.2, 7.5) ccw
  line L164 (41.2, 7.5) -> (41.2, 26)
  point P0 (85.4, 28.5)
  point P1 (47.15, 7.5)
  point P2 (19.7731, 1.7149)
  point P3 (78.617, 0)
  point P4 (80.0027, 0)
  point P5 (55.3909, 28.3)
  point P6 (55.7442, 27.1)
  point P7 (55.3896, 16.886)
  point P8 (55.2, 16.1835)
  point P9 (60.9311, 0)
  point P10 (63.617, 0)
  point P11 (18.783, 0)
  point P12 (19.0689, 0)
  point P13 (27.2, 16.1835)
  point P14 (27.0104, 16.886)
  point P15 (26.6558, 27.1)
  point P16 (27.0091, 28.3)
  point P17 (2.3973, 0)
  point P18 (3.783, 0)
  point P19 (57.7, 12.4676)
  point P20 (57.7, 10.7047)
  point P21 (57.7, 4.2953)
  point P22 (57.7, 0)
  point P23 (2.5571, 0.2767)
  point P24 (79.8429, 0.2767)
  point P25 (55.5333, 27.1)
  point P26 (55.2, 17.1)
  point P27 (28.2835, 15.1)
  point P28 (54.1165, 15.1)
  point P29 (62.2316, 0)
  point P30 (55.2, 17.1)
  point P31 (27.2, 28.3)
  point P32 (20.1684, 0)
  point P33 (58.9639, 6.925)
  point P34 (58.9639, 8.075)
  point P35 (35.3361, 8.075)
  point P36 (35.3361, 6.925)
  dimension "d244" = 3
  dimension "d259" = 1.3
  dimension "d260" = 4.5
  dimension "d261" = 14.5
  dimension "d262" = 9
  dimension "d263" = 0.025
  dimension "d264" = 0.475
  dimension "d265" = 2.775
  dimension "d266" = 0.95
  dimension "d267" = 0.1
  dimension "d268" = 3.85
  dimension "d269" = 3
  dimension "d270" = 28
  dimension "d271" = 12
  dimension "d273" = 180
  dimension "d274" = 180
  dimension "d276" = 4
  dimension "d277" = 15
  dimension "d278" = 7
  dimension "d279" = 24
  dimension "d280" = 130
  dimension "d283" = 15
  dimension "d285" = 7
  dimension "d286" = 120
  dimension "d289" = 28
  dimension "d290" = 15
  dimension "d291" = 2
  dimension "d292" = 1
  dimension "d293" = 3
  dimension "d294" = 2
  dimension "d295" = 1
  dimension "d296" = 3
  dimension "d297" = 2
  dimension "d298" = 3
  dimension "d299" = 1
  dimension "d300" = 5
  dimension "d301" = 3
  dimension "d302" = 1
  dimension "d303" = 2
  dimension "d304" = 2
  dimension "d305" = 2
  dimension "d306" = 2
  dimension "d307" = 0.2
  dimension "d311" = 15
  dimension "d312" = 15
  dimension "d313" = 7
  dimension "d314" = 8
  dimension "d315" = 5
  dimension "d316" = 1.6
  dimension "d317" = 1.2
  dimension "d318" = 1.2
  dimension "d323" = 1.3
  dimension "d324" = 1.016
  dimension "d326" = 0.1
  dimension "d327" = 7
  dimension "d328" = 7.2
  dimension "d333" = 18.5
  dimension "d334" = 18.5
  constraints: 328 end point, 44 point on circle, 36 symmetric about line, 28 parallel, 25 point on line, 24 centre point, 17 horizontal, 17 perpendicular, 9 midpoint, 8 tangent, 6 collinear, 4 coincident, 3 vertical, 2 equal length, 49 other
  measures "d244" distance of L6.end L5.end
  measures "d259" distance of L8.end L9.end
  measures "d260" distance of L7.end L8.end
  measures "d261" distance of L8.end L11.end
  measures "d262" diameter of A1
  measures "d263" distance of L16.end L17.end
  measures "d264" distance of L15.end L16.end
  measures "d265" distance of L20.end L21.end
  measures "d266" distance of L19.end L20.end
  measures "d267" distance between parallel lines of L14 L23
  measures "d268" diameter of A4
  measures "d269" distance of L25.start L25.end
  measures "d270" distance of L27.end L28.end
  measures "d271" distance of L26.end L27.end
  measures "d273" angle of L31 L32
  measures "d274" angle of L31 L33
  measures "d276" distance of L3.end L36.end
  measures "d277" distance of L36.end L37.end
  measures "d278" distance of L26.start L40.end
  measures "d279" distance of L40.end L41.end
  measures "d280" angle of L41 L40
  measures "d283" distance of L42.start L42.end
  measures "d285" distance of L41.end L43.end
  measures "d286" angle of L44 L45
  measures "d289" distance of L48.end L47.end
  measures "d290" distance of L47.end L46.end
  measures "d291" distance of L48.end L50.end
  measures "d292" distance of L53.end L52.end
  measures "d293" distance of L52.end L51.end
  measures "d294" distance of L28.end L55.end
  measures "d295" distance of L57.end L58.end
  measures "d296" distance of L56.end L57.end
  measures "d297" distance of L48.end L63.end
  measures "d298" distance of L66.end L65.end
  measures "d299" distance of L65.end L64.end
  measures "d300" distance of L65.end L69.start
  measures "d301" distance of L70.end L71.end
  measures "d302" distance of L69.end L70.end
  measures "d303" radius of A5
  measures "d304" radius of A6
  measures "d305" radius of A7
  measures "d306" radius of A8
  measures "d307" distance between parallel lines of L83 L90
  measures "d311" distance of L44.end L110.end
  measures "d312" distance of L41.end L111.end
  measures "d313" distance of L111.end point (19.773, 1.715)
  measures "d314" radius of A13
  measures "d315" radius of A14
  measures "d316" distance of L26.start L122.end
  measures "d317" distance between parallel lines of L41 L129
  measures "d318" distance between parallel lines of L116 L138
  measures "d323" distance of L142.end L141.end
  measures "d324" distance of L148.end L147.end
  measures "d326" distance between parallel lines of L21 L154
  measures "d327" diameter of A21
  measures "d328" diameter of A22
  measures "d333" distance of L31.start L162.end
  measures "d334" radius of A23
ref_plane "РабПлоскость5" through (0, 0, 88.4) normal (-1, 0, 0) x (0, 0, 1)
ref_plane "РабПлоскость6" through (0, 0, 44.2) normal (0, 0, -1) x (-1, 0, 0)
ref_plane "РабПлоскость7" through (-24.9, -28.5, 85.4) normal (1, 0, 0) x (0, 0, -1)
extrude "Выдавливание32" add sketch "Эскиз14" against normal blind 13.2 from surface at -2 contours L3 L153 L136 | L127 L151 L3 | L3 L118 L117 L116 L115 L94 A10 L139 L138 L137 L136 L153 | L136 L137 L152 L153 | L151 L127 L128 L129 L130 A11 L102 L40 L41 L43 L44 L3 | L151 L150 L128 L127 | L3 L120 A16 L119 A15 L121 A23 L92 L93 L94 L115 L116 L117 L118 | L44 L43 L41 L40 L102 L103 L104 A23 L114 A13 L112 A14 L113 L3 | L3 A20 L133 A19 L161 L160 L159 L132 A23 L121 A15 L119 A16 L120 | L3 A23 L161 A19 L133 A20 | L113 A14 L112 A13 L114 A23 L123 A17 L124 A18 L3 | A18 L124 A17 L123 A23 L3 | L3 L145 L163 | L163 L145 A2 L161 A23 | L130 L122 L60 L40 L102 A11 | A23 L159 A19 L161 | L161 A2 L159 A23 | L94 L93 L92 A23 L76 L75 L74 L115 | L40 L60 L61 L62 A23 L104 L103 L102 | L162 L144 L3 | A23 L123 L144 L162 | L145 A1 L161 A2 | A19 L159 L160 L161 | L161 A1 L159 A2 | A23 L132 A19 L159 | L159 A2 L145 L132 A23 | L74 L75 L76 A23 L27 L115 | L60 L122 L40 | L40 L29 A23 L62 L61 L60 | A23 L114 A12 L29 L123 | L145 A22 A1 | L159 A1 L145 A2 | L132 L27 A9 L121 A23 | L121 A9 L92 A23 | L27 A23 L29 L26 | A23 L104 A12 L114 | L145 A21 A22 | L121 L76 A23 L92 A9 | A9 L27 L121 | A23 L76 L27 | L27 A7 L28 L164 A23 | A23 L164 L28 A8 L29 | L29 L62 A23 | A23 L62 L114 A12 L104 | L29 A12 L28 | L114 L29 A12 | L145 A21 | L27 L28 A9 | A9 L28 A7 L27 | A8 L28 A12 L29 picked at (57.9479, 7.7958) picked at (57.7369, 7.238)
extrude "Выдавливание33" cut sketch "Эскиз14" against normal blind 12 from surface at -2 contours L3 L120 A16 L119 A15 L121 A23 L92 L93 L94 L115 L116 L117 L118 | L44 L43 L41 L40 L102 L103 L104 A23 L114 A13 L112 A14 L113 L3 | L121 A9 L92 A23 | A23 L104 A12 L114
extrude "Выдавливание31" cut sketch "Эскиз14" against normal blind 55.6 contours A10 L94 L115 L74 A6 L77 L78 L79 L88 L87 L86 L68 A5 L122 L130 A11 L101 L100 L99 L98 L97 L96 L95 | L130 L122 L60 L40 L102 A11 | L94 L93 L92 A23 L76 L75 L74 L115 | L40 L60 L61 L62 A23 L104 L103 L102 | L115 L26 L122 A5 L68 L86 L87 L88 L79 L78 L77 A6 L74 | L74 L75 L76 A23 L27 L115 | L60 L122 L40 | L40 L29 A23 L62 L61 L60 | L27 A23 L29 L26 | L121 L76 A23 L92 A9 | A9 L27 L121 | A23 L76 L27 | L27 A7 L28 L164 A23 | A23 L164 L28 A8 L29 | L29 L62 A23 | A23 L62 L114 A12 L104 | L114 L29 A12 | A9 L28 A7 L27 | A8 L28 A12 L29 | A9 L91 L90 L109 L108 L164 L28 L85 L83 L84 | L84 L83 L85 L28 | L164 L108 L107 L106 L105 A12 L28 L80 L81 L82 | L28 L82 L81 L80
extrude "Выдавливание34" cut sketch "Эскиз14" against normal blind 22.8 contours A23 L159 A19 L161 | L161 A2 L159 A23 | L145 A1 L161 A2 | A2 L24 L163 L13 A1 L145 | L24 A3 L162 A0 L13 L163 | A19 L159 L160 L161 | L161 A1 L159 A2 | L145 A22 A1 | A1 L13 L163 A4 L164 L14 L145 A22 | L13 A0 L162 A4 L163 | L159 A1 L145 A2 | A3 L156 A0 L162 | A22 L145 A21 | L145 A21 A22 | L163 L164 A4 | A4 L162 L163 | L145 A1 L14 L164 L23 A2 | L156 L155 L154 A3 L21 L20 L19 | A3 L19 A0 L156 | A0 L156 L157 L154 L14 L164 A4 L162 | A21 L145 | L145 A21 | A4 L164 L162 | A3 L21 A0 L19 | L19 L20 L21 A3 | A0 L22 L154 L157 L156 | L164 L14 A0 L154 A3 L23 | A0 L22 | A3 L154 A0 L21